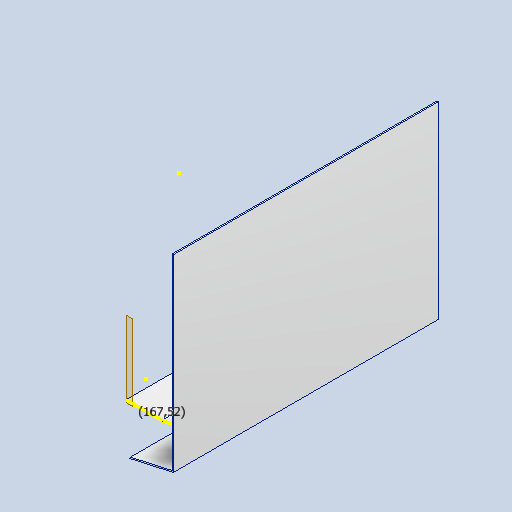
# Autodesk Inventor part: pokrywa
Saved by Autodesk Inventor 2023 (Build 270158000, 158)
## iProperties
Created: 2022-10-11
Part Number: pokrywa
Material: Aluminum 6061
Document SubType Name: Modeling
Designer: komputer
Density: 2.7 g/cm^3
Appearance: Aluminum - Flat
Author: komputer
Autodesk Inventor part; units mm, degrees
ref_plane "YZ Plane" through (0, 0, 0) normal (1, 0, 0) x (0, 1, 0)
ref_plane "XZ Plane" through (0, 0, 0) normal (0, 1, 0) x (-1, 0, 0)
ref_plane "XY Plane" through (0, 0, 0) normal (0, 0, 1) x (1, 0, 0)
sketch "Sketch1" plane through (0, 0, 0) normal (0, 0, 1) x (1, 0, 0)
  line L0 (-17.5, 7.6319) -> (17.5, -9.8679) projected
  line L1 (17.5, -9.8679) -> (17.5, -7.6319) projected
  line L2 (17.5, -7.6319) -> (-17.5, 9.8679) projected
  line L3 (-17.5, 9.8679) -> (-17.5, 7.6319) projected
  line L4 (-7.5, -29.4219) -> (-3.6225, -29.4219) projected
  arc A0 (-1.9153, -30.38) -> (-3.6225, -29.4219) centre (-3.6225, -31.4219) ccw projected
  line L5 (-1.9153, -30.38) -> (2.2072, -37.135) projected
  arc A1 (2.5, -38.1769) -> (2.2072, -37.135) centre (0.5, -38.1769) ccw projected
  line L6 (2.5, -38.1769) -> (2.5, -47.4219) projected
  arc A2 (0.5, -49.4219) -> (2.5, -47.4219) centre (0.5, -47.4219) ccw projected
  line L7 (0.5, -49.4219) -> (-7.5, -49.4219) projected
  line L8 (-7.5, -49.4219) -> (-7.5, -29.4219) projected
  spline S0 degree 3 poles (6.0485, -14.3337) (6.0213, -14.5971) (5.9428, -14.8528) (5.6929, -15.3183) (5.524, -15.5241) (5.1467, -15.8339) (4.9505, -15.9462) (4.5292, -16.1007) (4.3073, -16.1418) (4.0832, -16.1449) knots 0 0 0 0 0.079442 0.079442 0.158531 0.158531 0.225919 0.225919 0.293184 0.293184 0.293184 0.293184 projected
  line L9 (6.0485, -14.3337) -> (6.563, -9.3583) projected
  line L10 (6.563, -9.3583) -> (6.8849, -5.9915) projected
  arc A3 (6.8849, -5.9915) -> (5.7884, -4.0122) centre (4.894, -5.8011) ccw projected
  line L11 (-17.5, 7.6319) -> (5.7884, -4.0122) projected
  line L12 (-17.5, -57.5975) -> (-17.5, 7.6319) projected
  arc A4 (-4.376, -58.868) -> (-17.5, -57.5975) centre (-12.5, -74.368) ccw projected
  arc A5 (1.8324, -81.8643) -> (-4.376, -58.868) centre (-12.5, -73.3975) ccw projected
  line L13 (17.5, -78.3975) -> (17.5, -28.6365) projected
  ellipse E0 centre (15.5, -28.6365) end of major axis (15.5, -26.6191) minor radius 2 (17.5, -28.6365) -> (15.6888, -26.6281) ccw projected
  line L14 (15.6888, -26.6281) -> (3.1949, -25.4333) projected
  line L15 (3.1949, -25.4333) -> (4.0832, -16.1449) projected
  circle A6 centre (12, -52.3461) radius 1.25 projected
  circle A7 centre (-5.3255, -52.3461) radius 1.25 projected
  line L16 (14, -34.918) -> (10, -34.918) projected
  line L17 (14, -41.318) -> (14, -34.918) projected
  line L18 (10, -41.318) -> (14, -41.318) projected
  line L19 (10, -34.918) -> (10, -41.318) projected
  line L20 (-13.7851, -31.6782) -> (-9.7851, -31.6782) projected
  line L21 (-13.7851, -25.2782) -> (-13.7851, -31.6782) projected
  line L22 (-9.7851, -25.2782) -> (-13.7851, -25.2782) projected
  line L23 (-9.7851, -31.6782) -> (-9.7851, -25.2782) projected
  circle A8 centre (-7.1425, -17.0027) radius 1.25 projected
  line L24 (-19.5, -83.5975) -> (-17.5, -83.5975) projected
  line L25 (-17.5, -57.5975) -> (-17.5, -83.5975) projected
  line L26 (-19.5, -57.5975) -> (-17.5, -57.5975) projected
  line L27 (-19.5, -57.5975) -> (-19.5, -83.5975) projected
  line L28 (-12.5, -83.5975) -> (-17.5, -83.5975) projected
  arc A9 (-12.5, -83.5975) -> (-6.9024, -81.9243) centre (-12.5, -73.3975) ccw projected
  line L29 (17.5, -7.6319) -> (18, -7.6319)
  line L30 (18, -7.6319) -> (18, -79.7438)
  line L31 (18, -79.7438) -> (17.5, -79.7438)
  line L32 (17.5, -79.7438) -> (17.5, -7.6319)
  line L33 (-6, -67.7722) -> (-6, -79.3975) projected
  line L34 (-12.5, -83.5975) -> (-17.5, -83.5975) projected
  arc A10 (-12.5, -83.5975) -> (-6.9024, -81.9243) centre (-12.5, -73.3975) ccw projected
  arc A11 (-6.9024, -81.9243) -> (-6, -80.2524) centre (-8, -80.2524) ccw projected
  line L35 (-6, -79.3975) -> (-6, -67.7722) projected
  line L36 (-6, -80.2524) -> (-6, -79.3975) projected
  line L37 (-19.5, -83.5975) -> (-6, -83.5975)
  line L38 (-6, -83.5975) -> (-6, -84.0975)
  line L39 (-6, -84.0975) -> (-19.5, -84.0975)
  line L40 (-19.5, -84.0975) -> (-19.5, -83.5975)
  line L41 (-6, -83.5975) -> (17.5, -78.3975)
  line L42 (16.4042, -78.64) -> (16.5122, -79.1281)
  line L43 (-3.7701, -83.1041) -> (-3.6621, -83.5922)
  line L44 (16.5122, -79.1281) -> (-3.6621, -83.5922)
  line L45 (16.5122, -79.1281) -> (21.5032, -78.0238)
  line L46 (-3.6621, -83.5922) -> (-17.5, -86.6542)
  line L47 (-6, -84.0975) -> (-5.7395, -84.0975)
  circle A12 centre (-12.5, -73.3975) radius 16.6465
  line L48 (1.8324, -81.8643) -> (17.5, -78.3975) projected
  point P0 (0, 0)
  point P1 (1.8324, -81.8643)
  point P2 (1.4649, -82.4578)
  point P3 (18, -78.7989)
  dimension "d0" = 0.5
  dimension "d1" = 0.5
  dimension "d4" = 0.5
  dimension "d5" = 0.5
  constraints: 30 end point, 4 parallel, 4 perpendicular, 3 horizontal, 2 point on line, 1 centre point, 1 coincident, 1 concentric, 1 other
  measures "d0" distance of L30.end L31.end
  measures "d1" distance of L37.end L38.end
  measures "d4" distance of L42.start L42.end
  measures "d5" distance of L43.start L43.end
extrude "Extrusion1" add sketch "Sketch1" against normal blind 100 contours L1 L29 L30 L45 L32 L13 | L32 L45 L42 L41 | L41 L42 L44 A12
ref_plane "Work Plane1" through (-19.5, -57.5975, -20) normal (0, 0, 1) x (1, 0, 0)
sketch "Sketch2" plane through (-19.5, -57.5975, -20) normal (0, 0, 1) x (1, 0, 0)
  line L0 (0, -26) -> (2, -26) projected
  line L1 (2, 0) -> (2, -26) projected
  line L2 (0, 0) -> (2, 0) projected
  line L3 (0, 0) -> (0, -26) projected
  line L4 (7, -26) -> (2, -26) projected
  arc A0 (7, -26) -> (12.5976, -24.3269) centre (7, -15.8) ccw projected
  line L5 (13.5, -21.8) -> (13.5, -10.1747) projected
  line L6 (0, -26) -> (13.5546, -26)
  line L7 (13.5546, -26) -> (13.5546, -26.5)
  line L8 (13.5546, -26.5) -> (0, -26.5)
  line L9 (0, -26.5) -> (0, -26)
  line L10 (37.5, -21.2015) -> (20.9649, -24.8603) projected
  line L11 (13.5546, -26.5) -> (20.9649, -24.8603)
  line L12 (20.9649, -24.8603) -> (37.5, -21.2015) projected
  line L13 (37.5, -21.2015) -> (37.5, 49.9656) projected
  line L14 (37.5, 49.9656) -> (37, 49.9656) projected
  line L15 (37, 49.9656) -> (37, -20.8) projected
  line L16 (37, -20.8) -> (21.3324, -24.2669) projected
  arc A1 (20.9649, -24.8603) -> (21.3324, -24.2669) centre (7, -15.8) ccw projected
  arc A2 (20.9649, -24.8603) -> (21.3324, -24.2669) centre (7, -15.8) ccw projected
  line L17 (21.3324, -24.2669) -> (13.5, -26)
  point P0 (19.5, 57.5975)
  dimension "d8" = 0.5
  constraints: 12 end point, 2 parallel, 1 collinear, 1 horizontal, 1 perpendicular, 1 point on line
  measures "d8" distance of L6.end L7.end
extrude "Extrusion2" add sketch "Sketch2" against normal blind 60 contours L0 L4 L6 L7 L8 L9 | L7 L6 L17 A1 L11
sketch "Sketch3" plane through (-19.5, -57.5975, -20) normal (0, 0, 1) x (1, 0, 0)
  line L0 (0, -26.5) -> (13.5546, -26.5) projected
  line L1 (13.5546, -26.5) -> (20.9649, -24.8603) projected
  arc A0 (20.9649, -24.8603) -> (21.3324, -24.2669) centre (7, -15.8) ccw projected
  line L2 (21.3324, -24.2669) -> (13.5, -26) projected
  line L3 (13.5, -26) -> (0, -26) projected
  line L4 (0, -26) -> (0, -26.5) projected
  point P0 (19.5, 57.5975)
  dimension "d11" = 167.523
  measures "d11" angle of L3 L2
body "Solid1"
